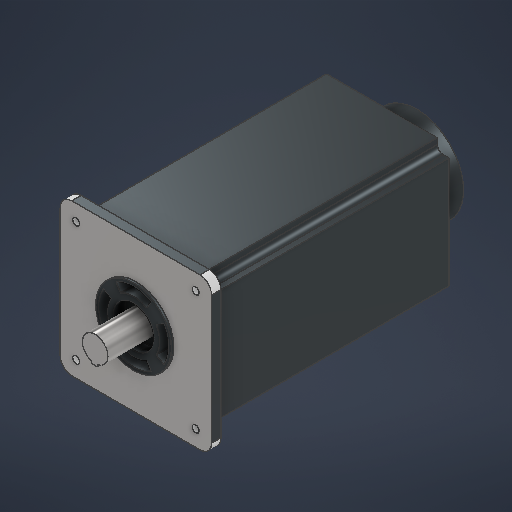
# Autodesk Inventor part: SERVOMOTOR-1KW
Saved by Autodesk Inventor 2025.3 (Build 293356030, 356C)
## iProperties
Created: 2025-09-01
Part Number: SERVOMOTOR-1KW
Material: Generic
Document SubType Name: Modeling
Designer: lstk1ng
Density: 1 g/cm^3
Appearance: Default
Author: lstk1ng
Autodesk Inventor part; units mm, degrees
ref_plane "YZ Plane" through (0, 0, 0) normal (1, 0, 0) x (0, 1, 0)
ref_plane "XZ Plane" through (0, 0, 0) normal (0, 1, 0) x (-1, 0, 0)
ref_plane "XY Plane" through (0, 0, 0) normal (0, 0, 1) x (1, 0, 0)
sketch "Sketch1" plane through (0, 0, 0) normal (0, 0, 1) x (1, 0, 0)
  line L0 (-55, 65) -> (55, 65)
  line L1 (65, 55) -> (65, -55)
  line L2 (55, -65) -> (-55, -65)
  line L3 (-65, -55) -> (-65, 55)
  circle A0 centre (0, 0) radius 32.5
  arc A1 (55, -65) -> (65, -55) centre (55, -55) ccw
  arc A2 (-65, -55) -> (-55, -65) centre (-55, -55) ccw
  arc A3 (-55, 65) -> (-65, 55) centre (-55, 55) ccw
  arc A4 (65, 55) -> (55, 65) centre (55, 55) ccw
  point P0 (-65, 65)
  point P1 (65, 65)
  point P2 (-65, -65)
  point P3 (65, -65)
  point P4 (-65, 0)
  point P5 (0, -65)
  dimension "d2" = 65
  dimension "d64" = 10
  constraints: 8 end point, 8 point on circle, 8 point on line, 8 tangent, 5 centre point, 3 equal radius, 2 midpoint, 2 parallel, 1 coincident, 1 horizontal, 1 horizontal alignment, 1 perpendicular, 1 vertical alignment
  measures "d2" diameter of A0
  measures "d64" radius of A1
extrude "Extrusion1" add sketch "Sketch1" along normal blind 8
sketch "Sketch2" plane through (0, 0, 0) normal (0, 0, 1) x (1, 0, 0)
  circle A0 centre (0, 0) radius 32.5
  line L0 (11.25, 19.4856) -> (15, 25.9808)
  line L1 (0, 0) -> (30, 0) construction
  line L2 (-11.25, 19.4856) -> (-15, 25.9808)
  line L3 (0, 0) -> (30, 0) construction
  line L4 (-19.4856, -11.25) -> (-25.9808, -15)
  line L5 (-19.4856, 11.25) -> (-25.9808, 15)
  line L6 (11.25, -19.4856) -> (15, -25.9808)
  line L7 (-11.25, -19.4856) -> (-15, -25.9808)
  line L8 (19.4856, 11.25) -> (25.9808, 15)
  line L9 (19.4856, -11.25) -> (25.9808, -15)
  arc A1 (15, 25.9808) -> (-15, 25.9808) centre (0, 0) ccw
  arc A2 (25.9808, -15) -> (25.9808, 15) centre (0, 0) ccw
  arc A3 (-25.9808, 15) -> (-25.9808, -15) centre (0, 0) ccw
  arc A4 (-15, -25.9808) -> (15, -25.9808) centre (0, 0) ccw
  circle A5 centre (0, 0) radius 17.5
  arc A6 (-19.4856, 11.25) -> (-19.4856, -11.25) centre (0, 0) ccw
  arc A7 (-11.25, -19.4856) -> (11.25, -19.4856) centre (0, 0) ccw
  arc A8 (19.4856, -11.25) -> (19.4856, 11.25) centre (0, 0) ccw
  arc A9 (11.25, 19.4856) -> (-11.25, 19.4856) centre (0, 0) ccw
  dimension "d15" = 60
  dimension "d16" = 120
  dimension "d19" = 360
  dimension "d21" = 35
  constraints: 20 end point, 16 point on circle, 10 centre point, 4 coincident, 2 horizontal, 25 other
  measures "d15" angle of L1 L0
  measures "d16" angle of L3 L2
  measures "d21" diameter of A5
extrude "Extrusion2" add sketch "Sketch2" along normal blind 10
sketch "Sketch3" plane through (0, 0, 0) normal (0, 0, -1) x (-1, 0, 0)
  line L0 (47.5, -57.5) -> (-47.5, -57.5)
  line L1 (-57.5, -47.5) -> (-57.5, 47.5)
  line L2 (-47.5, 57.5) -> (47.5, 57.5)
  line L3 (57.5, 47.5) -> (57.5, -47.5)
  line L4 (57.5, -57.5) -> (-57.5, 57.5) construction
  line L5 (-57.5, -57.5) -> (57.5, 57.5) construction
  line L6 (57.5, 47.5) -> (47.5, 47.5)
  line L7 (47.5, 47.5) -> (47.5, 57.5)
  line L8 (-61.2408, 0) -> (60.2976, 0)
  line L9 (0, 62.5016) -> (0, -60.5434)
  line L10 (57.5, -47.5) -> (47.5, -47.5)
  line L11 (47.5, -47.5) -> (47.5, -57.5)
  line L12 (-57.5, 47.5) -> (-47.5, 47.5)
  line L13 (-47.5, 47.5) -> (-47.5, 57.5)
  line L14 (-57.5, -47.5) -> (-47.5, -47.5)
  line L15 (-47.5, -47.5) -> (-47.5, -57.5)
  point P0 (0, 0)
  dimension "d61" = 115
  constraints: 32 end point, 9 symmetric about line, 3 perpendicular, 2 midpoint, 2 parallel, 1 horizontal, 1 point on line, 1 vertical
  measures "d61" distance of L5.start L4.end
extrude "Extrusion3" add sketch "Sketch3" along normal blind 203
fillet "Fillet1" radius 5 4 edges at (-47.5, -47.5, -101.5) (-47.5, 47.5, -101.5) (47.5, 47.5, -101.5) (47.5, -47.5, -101.5)
sketch "Sketch4" plane through (0, 0, -203) normal (0, 0, -1) x (-1, 0, 0)
  arc A0 (34.641, 20) -> (34.641, -20) centre (0, 0) ccw
  line L0 (34.641, 20) -> (59.641, 20)
  line L1 (59.641, 20) -> (59.641, -20)
  line L2 (59.641, -20) -> (34.641, -20)
  dimension "d34" = 25
  dimension "d35" = 40
  constraints: 6 end point, 2 perpendicular, 2 point on circle, 1 centre point, 1 coincident, 1 horizontal
  measures "d34" distance of L0.start L0.end
  measures "d35" distance of L0.end L1.end
extrude "Extrusion4" add sketch "Sketch4" along normal blind 30
sketch "Sketch6" plane through (0, 0, 0) normal (0, 0, 1) x (1, 0, 0)
  arc A0 (1.9444, -10.8268) -> (-3.0556, -10.5671) centre (0, 0) ccw
  line L0 (-0.5556, -10.9213) -> (-0.5556, -9.9213) construction
  line L1 (-0.5556, -9.9213) -> (-3.0556, -9.9213) construction
  line L2 (-3.0556, -9.9213) -> (-0.5556, -9.9213) construction
  line L3 (1.9444, -9.9213) -> (1.9444, -12.4213)
  line L4 (1.9444, -12.4213) -> (-3.0556, -12.4213)
  line L5 (-3.0556, -12.4213) -> (-3.0556, -9.9213)
  dimension "d44" = 22
  dimension "d45" = 1
  dimension "d46" = 2.5
  dimension "d47" = 5
  dimension "d48" = 2.5
  constraints: 12 end point, 2 horizontal, 2 parallel, 2 point on circle, 2 point on line, 1 centre point, 1 coincident, 1 perpendicular, 1 vertical
  measures "d44" diameter of A0
  measures "d45" distance of L0.end L0.start
  measures "d46" distance of L0.end L1.end
  measures "d47" distance of L3.end L4.end
  measures "d48" distance of L3.start L3.end
extrude "Extrusion6" add sketch "Sketch6" along normal blind 43
sketch "Sketch7" plane through (0, 0, 8) normal (0, 0, 1) x (1, 0, 0)
  circle A0 centre (0, 0) radius 17.5 projected
  circle A1 centre (0, 0) radius 72.5 construction
  arc A2 (65, 55) -> (55, 65) centre (55, 55) ccw projected
  line L0 (0, 0) -> (55, 55) construction
  circle A3 centre (51.2652, 51.2652) radius 3
  arc A4 (1.9444, -10.8268) -> (-3.0556, -10.5671) centre (0, 0) ccw projected
  line L1 (0, 0) -> (0, -48.5736)
  line L2 (0, 0) -> (55, 0)
  circle A5 centre (51.2652, -51.2652) radius 3
  circle A6 centre (-51.2652, 51.2652) radius 3
  circle A7 centre (-51.2652, -51.2652) radius 3
  dimension "d63" = 145
  dimension "d65" = 6
  constraints: 6 end point, 4 centre point, 3 symmetric about line, 1 coincident, 1 horizontal, 1 point on line, 1 vertical, 6 other
  measures "d65" diameter of A3
extrude "Extrusion7" cut sketch "Sketch7" against normal up to surface (8 mm away) contours A3 | A5 | A6 | A7
body "Solid1"
